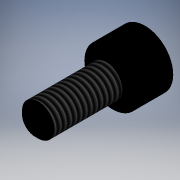
# Autodesk Inventor part: 11-5512_
Saved by Autodesk Inventor 2017.3 (Build 213256000, 256)
## iProperties
Part Number: 11-5512_
Material: Generic
Catalog Web Link: www.cadenas.de
Description: 11-5512, 11-5516, 19-6520, 13184, 11-5312_-Bolt
Vendor: 8020
Document SubType Name: Modeling
Designer: partserver
Manufacturer: 8020
Mass: 0.47703 g
Surface Area: 4.95509 cm^2
Volume: 0.47703 cm^3
Density: 1 g/cm^3
Appearance: PSOLRGB-0-0-0
Category: PARTsolutions
Company: 8020
Title: 11-5512_
Author: Cadenas PARTsolutions
Comments: Bolt
PSOL_IDENT_0: {$CADENAS_DATA\23d-libs\8020\metric\fastening_options\11_5516.prj},192 {VTYP=3D},{NB=11-5512_},{LINA=
PSOL_IDENT_1: 11-5512_},{NN=11-5512, 11-5516, 19-6520, 13184, 11-5312_},{DATE=31.07.2020 09:21:25},{GEOMDATE=18.12
PSOL_IDENT_2: .2018 15:13:00},{VERSION=},{LINEID=10},{WBVAR=},{WBNUMERIC=}  {NB=11-5512_},{LINA=11-5512_},{KT=DUMM
PSOL_IDENT_3: Y},{PN=11-5512},{A=5.000},{L=12.000},{D=8.720},{M=5.000},{WF=4.000},{T=4.000},{NO=1},{X=0.000},{D1=0
PSOL_IDENT_4: .000},{COL=0,0,0}
NB: 11-5512_
NN: 11-5512, 11-5516, 19-6520, 13184, 11-5312_
NT: Bolt
NBSYN: $PN._
LINA: 11-5512_
CATALOG: 80/20
PN: 11-5512
A: 5
L: 12
D: 8.72
M: 5
WF: 4
T: 4
NO: 1
X: 0
D1: 0
SUPPLIER: 8020
ARTICLENO: 11-5512_
BOMINFO: 11-5512_
CREATOR: CADENAS GmbH
Autodesk Inventor part; units mm, degrees
sketch "Sketch_1" plane through (0, 0, 0) normal (0, 0, 1) x (1, 0, 0)
  line L0 (0, -12) -> (0, 5)
  line L1 (0, 5) -> (4.36, 5)
  line L2 (4.36, 5) -> (4.36, 0)
  line L3 (4.36, 0) -> (2.5, 0)
  line L4 (2.5, 0) -> (2.5, -11.5095)
  line L5 (2.5, -11.5095) -> (2.0095, -12)
  line L6 (2.0095, -12) -> (0, -12)
  line L7 (0, -12) -> (0, 5)
  constraints: 16 end point
revolve "Revolution1" add sketch "Sketch_1" angle 360 about axis through (0, -12, 0) along (0, -1, 0)
thread "Thread1" size "M5x0.8" class "6g" standard "ISO Metric profile" length 10.5095
sketch "Sketch_2" plane through (0, 5, 0) normal (0, 1, 0) x (1, 0, 0)
  line L0 (-2, -1.1547) -> (0, -2.3094)
  line L1 (0, -2.3094) -> (2, -1.1547)
  line L2 (2, -1.1547) -> (2, 1.1547)
  line L3 (2, 1.1547) -> (0, 2.3094)
  line L4 (0, 2.3094) -> (-2, 1.1547)
  line L5 (-2, 1.1547) -> (-2, -1.1547)
  constraints: 12 end point
extrude "Extrusion1" cut sketch "Sketch_2" against normal blind 4
ref_plane "1_XY" through (0, 0, 0) normal (0, 1, 0) x (1, 0, 0)
ref_plane "1_YZ" through (0, 0, 0) normal (1, 0, 0) x (0, 0, -1)
ref_plane "1_ZX" through (0, 0, 0) normal (0, 0, -1) x (0, 1, 0)
ref_plane "2_XY" through (0, -12, 0) normal (0, 1, 0) x (1, 0, 0)
ref_plane "2_YZ" through (0, -12, 0) normal (1, 0, 0) x (0, 0, -1)
ref_plane "2_ZX" through (0, -12, 0) normal (0, 0, -1) x (0, 1, 0)
body "Solid1"
